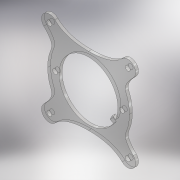
# Autodesk Inventor part: YawMotorPlate
Saved by Autodesk Inventor 2018 (Build 220112000, 112)
## iProperties
Created: 2018-03-25
Part Number: YawMotorPlate
Material: Glass
Document SubType Name: Modeling
Designer: mansu
Density: 2.18 g/cm^3
Appearance: Clear Clear
Author: mansu
Autodesk Inventor part; units mm, degrees
ref_plane "YZ Plane" through (0, 0, 0) normal (1, 0, 0) x (0, 1, 0)
ref_plane "XZ Plane" through (0, 0, 0) normal (0, 1, 0) x (-1, 0, 0)
ref_plane "XY Plane" through (0, 0, 0) normal (0, 0, 1) x (1, 0, 0)
sketch "Sketch1" plane through (0, 0, 0) normal (0, 1, 0) x (-1, 0, 0)
  arc A0 (-27.704, 11.5104) -> (-27.6923, -11.5384) centre (0, 0) ccw
  line L0 (0, 0) -> (-57.7769, 0) construction
  circle A1 centre (34.141, 0) radius 2.5
  circle A2 centre (-34.141, 0) radius 2.5
  line L1 (34.141, 0) -> (-34.141, 0) construction
  line L2 (40, -40) -> (-40, -40) construction
  line L3 (-40, -40) -> (-40, 40) construction
  line L4 (-40, 40) -> (40, 40) construction
  line L5 (40, 40) -> (40, -40) construction
  line L6 (40, -40) -> (-40, 40) construction
  line L7 (-40, -40) -> (40, 40) construction
  circle A3 centre (40, -40) radius 2.5
  circle A4 centre (-40, -40) radius 2.5
  circle A5 centre (40, 40) radius 2.5
  circle A6 centre (-40, 40) radius 2.5
  arc A7 (-45.6569, -34.3431) -> (-34.3431, -45.6569) centre (-40, -40) ccw
  line L8 (-34.3431, -45.6569) -> (-45.6569, -34.3431) construction
  line L9 (-34.3431, -45.6569) -> (-23.6863, -35) construction
  line L10 (-23.6863, -35) -> (0, -35) construction
  spline S0 degree 2 poles (-34.3431, -45.6569) (-23.6863, -35) (0, -35) knots 1 1 1 2 2 2
  arc A8 (-25.3751, 16.0032) -> (-27.704, 11.5104) centre (0, 0) ccw
  line L11 (-45.6569, -34.3431) -> (-35, -23.6863) construction
  line L12 (-35, -23.6863) -> (-35, -18) construction
  line L13 (-35, -18) -> (-41.641, -18) construction
  line L14 (-41.641, -18) -> (-41.641, 0) construction
  spline S1 degree 4 poles (-45.6569, -34.3431) (-35, -23.6863) (-35, -18) (-41.641, -18) (-41.641, 0) knots 1 1 1 1 1 2 2 2 2 2
  arc A9 (-34.3431, 45.6569) -> (-45.6569, 34.3431) centre (-40, 40) ccw
  line L15 (-34.3431, 45.6569) -> (-23.6863, 35) construction
  line L16 (-23.6863, 35) -> (0, 35) construction
  spline S2 degree 2 poles (-34.3431, 45.6569) (-23.6863, 35) (0, 35) knots 1 1 1 2 2 2
  line L17 (-45.6569, 34.3431) -> (-35, 23.6863) construction
  line L18 (-35, 23.6863) -> (-35, 18) construction
  line L19 (-35, 18) -> (-41.641, 18) construction
  line L20 (-41.641, 18) -> (-41.641, 0) construction
  spline S3 degree 4 poles (-45.6569, 34.3431) (-35, 23.6863) (-35, 18) (-41.641, 18) (-41.641, 0) knots 1 1 1 1 1 2 2 2 2 2
  line L21 (0, 0) -> (0, -30) construction
  arc A10 (34.3431, -45.6569) -> (45.6569, -34.3431) centre (40, -40) ccw
  line L22 (34.3431, -45.6569) -> (23.6863, -35) construction
  line L23 (23.6863, -35) -> (0, -35) construction
  spline S4 degree 2 poles (34.3431, -45.6569) (23.6863, -35) (0, -35) knots 1 1 1 2 2 2
  line L24 (45.6569, -34.3431) -> (35, -23.6863) construction
  line L25 (35, -23.6863) -> (35, -18) construction
  line L26 (35, -18) -> (41.641, -18) construction
  line L27 (41.641, -18) -> (41.641, 0) construction
  spline S5 degree 4 poles (45.6569, -34.3431) (35, -23.6863) (35, -18) (41.641, -18) (41.641, 0) knots 1 1 1 1 1 2 2 2 2 2
  arc A11 (45.6569, 34.3431) -> (34.3431, 45.6569) centre (40, 40) ccw
  spline S6 degree 4 poles (45.6569, 34.3431) (35, 23.6863) (35, 18) (41.641, 18) (41.641, 0) knots 1 1 1 1 1 2 2 2 2 2
  spline S7 degree 2 poles (34.3431, 45.6569) (23.6863, 35) (0, 35) knots 1 1 1 2 2 2
  line L28 (45.6569, 34.3431) -> (35, 23.6863) construction
  line L29 (35, 23.6863) -> (35, 18) construction
  line L30 (35, 18) -> (41.641, 18) construction
  line L31 (41.641, 18) -> (41.641, 0) construction
  line L32 (34.3431, 45.6569) -> (23.6863, 35) construction
  line L33 (23.6863, 35) -> (0, 35) construction
  line L34 (-25.3913, -15.9775) -> (-21.9327, -14.1847)
  line L35 (-21.9327, -14.1847) -> (-24.2337, -9.7457)
  line L36 (-24.2337, -9.7457) -> (-27.6923, -11.5384)
  line L37 (0, 0) -> (-23.0832, -11.9652) construction
  arc A12 (-27.6923, -11.5384) -> (-25.3913, -15.9775) centre (0, 0) ccw construction
  arc A13 (-25.3913, -15.9775) -> (-25.3751, 16.0032) centre (0, 0) ccw
  point P0 (-36.641, 0)
  point P1 (-30, 0)
  dimension "d0" = 60
  dimension "d4" = 5
  dimension "d5" = 68.282
  dimension "d6" = 80
  dimension "d7" = 80
  dimension "d8" = 5
  dimension "d9" = 5
  dimension "d10" = 5
  dimension "d11" = 5
  dimension "d12" = 8
  dimension "d13" = 45
  dimension "d14" = 5
  dimension "d15" = 5
  dimension "d16" = 5
  dimension "d17" = 18
  dimension "d20" = 5
  dimension "d21" = 26
  dimension "d22" = 27.4
  constraints: 28 end point, 23 symmetric about line, 22 point on circle, 13 centre point, 6 midpoint, 5 coincident, 5 perpendicular, 4 point on line, 3 horizontal, 3 horizontal alignment, 3 parallel, 3 vertical, 2 tangent, 2 vertical alignment, 1 collinear, 1 concentric, 30 other
  measures "d0" diameter of A0
  measures "d4" diameter of A1
  measures "d5" distance of L1.start L1.end
  measures "d6" distance of L3.end L4.end
  measures "d7" distance of L2.end L3.end
  measures "d8" diameter of A3
  measures "d9" diameter of A4
  measures "d10" diameter of A5
  measures "d11" diameter of A6
  measures "d12" radius of A7
  measures "d13" angle of L2 L8
  measures "d14" distance of L10.end L21.end
  measures "d15" distance from line of point (-30, 0) L12
  measures "d16" distance from line of point (-36.641, 0) L14
  measures "d17" distance of L13.end L14.end
  measures "d20" distance of L34.end L35.end
  measures "d21" distance of L21.start L37.end
  measures "d22" angle of L37 L0
extrude "Extrusion1" add sketch "Sketch1" along normal blind 3
body "Solid1"
